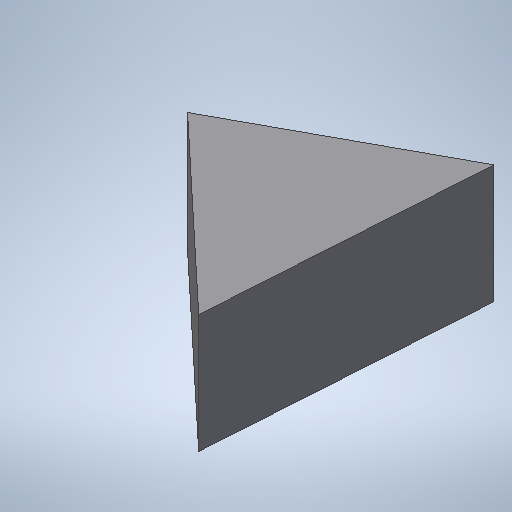
# Autodesk Inventor part: Triangle
Saved by Autodesk Inventor 2027 (Build 310192060, 192F)
## iProperties
Created: 2026-06-18
Part Number: Triangle
Material: Generisch
Document SubType Name: Modeling
Designer: tobia
Density: 1 g/cm^3
Appearance: Vorgabe
Author: tobia
Title: Test1
Autodesk Inventor part; units mm, degrees
ref_plane "YZ Plane" through (0, 0, 0) normal (1, 0, 0) x (0, 1, 0)
ref_plane "XZ Plane" through (0, 0, 0) normal (0, 1, 0) x (-1, 0, 0)
ref_plane "XY Plane" through (0, 0, 0) normal (0, 0, 1) x (1, 0, 0)
sketch "Sketch1" plane through (0, 0, 0) normal (0, 1, 0) x (-1, 0, 0)
  line L0 (-3.4492, 11.4342) -> (11.7965, -2.8664)
  line L1 (11.7965, -2.8664) -> (-4.9611, -11.9697)
  line L2 (-4.9611, -11.9697) -> (-3.4492, 11.4342)
  point P0 (0, 0)
  constraints: 6 end point
extrude "Extrusion1" add sketch "Sketch1" along normal blind 10
body "Solid1"
